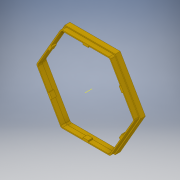
# Autodesk Inventor part: Cover v1
Saved by Autodesk Inventor 2019 (Build 230136000, 136)
## iProperties
Created: 2021-07-14
Part Number: Cover v1
Material: Generic
Document SubType Name: Modeling
Designer: Lix
Density: 1 g/cm^3
Appearance: Gold
d0: 175,000 mm
d1: 2,000 mm
d2: 0,00 deg
d15: 2,000 mm
d16: 2,000 mm
d17: 10,000 mm
d18: 0,00 deg
d19: 4,000 mm
d20: 7,000 mm
d21: 0,00 deg
d22: 10,000 mm
d23: 4,000 mm
d24: 10,000 mm
d25: 3,300 mm
d26: 6,500 mm
d27: 0,00 deg
d28: 4,000 mm
d29: 3,000 mm
d31: 0,00 deg
d32: 6,000 ul
d33: 360,00 deg
Author: Lix
Autodesk Inventor part; units mm, degrees
ref_plane "YZ Plane" through (0, 0, 0) normal (1, 0, 0) x (0, 1, 0)
ref_plane "XZ Plane" through (0, 0, 0) normal (0, 1, 0) x (-1, 0, 0)
ref_plane "XY Plane" through (0, 0, 0) normal (0, 0, 1) x (1, 0, 0)
sketch "Sketch1" plane through (0, 0, 0) normal (0, 0, 1) x (1, 0, 0)
  line L0 (50.5181, -87.5) -> (-50.5181, -87.5)
  line L1 (-50.5181, -87.5) -> (-101.0363, 0)
  line L2 (-101.0363, 0) -> (-50.5181, 87.5)
  line L3 (-50.5181, 87.5) -> (50.5181, 87.5)
  line L4 (50.5181, 87.5) -> (101.0363, 0)
  line L5 (101.0363, 0) -> (50.5181, -87.5)
  point P0 (0, 0)
  point P1 (0, 0)
  dimension "d0" = 175
  constraints: 12 end point, 1 coincident, 1 horizontal, 13 other
  measures "d0" distance between parallel lines of L4 L1
extrude "Extrusion1" add sketch "Sketch1" along normal blind 2
sketch "Sketch5" plane through (0, 0, 2) normal (0, 0, 1) x (1, 0, 0)
  line L0 (-50.5181, -87.5) -> (50.5181, -87.5) projected
  line L1 (50.5181, -87.5) -> (101.0363, 0) projected
  line L2 (101.0363, 0) -> (50.5181, 87.5) projected
  line L3 (50.5181, 87.5) -> (-50.5181, 87.5) projected
  line L4 (-50.5181, 87.5) -> (-101.0363, 0) projected
  line L5 (-101.0363, 0) -> (-50.5181, -87.5) projected
  line L6 (-98.7269, 0) -> (-49.3634, 85.5)
  line L7 (-49.3634, 85.5) -> (49.3634, 85.5)
  line L8 (49.3634, 85.5) -> (98.7269, 0)
  line L9 (98.7269, 0) -> (49.3634, -85.5)
  line L10 (49.3634, -85.5) -> (-49.3634, -85.5)
  line L11 (-49.3634, -85.5) -> (-98.7269, 0)
  line L12 (-96.4175, 0) -> (-48.2087, 83.5)
  line L13 (-48.2087, 83.5) -> (48.2087, 83.5)
  line L14 (48.2087, 83.5) -> (96.4175, 0)
  line L15 (96.4175, 0) -> (48.2087, -83.5)
  line L16 (48.2087, -83.5) -> (-48.2087, -83.5)
  line L17 (-48.2087, -83.5) -> (-96.4175, 0)
  point P0 (0, 0)
  dimension "d15" = 2
  dimension "d16" = 2
  constraints: 24 end point, 10 other
  measures "d15" distance between parallel lines of L4 L6
  measures "d16" distance between parallel lines of L11 L17
extrude "Extrusion5" add sketch "Sketch5" along normal blind 10 contours L6 L7 L8 L9 L10 L11
sketch "Sketch7" plane through (0, 0, 2) normal (0, 0, 1) x (1, 0, 0)
  line L0 (48.2087, 83.5) -> (-48.2087, 83.5) projected
  line L1 (-48.2087, 83.5) -> (-96.4175, 0) projected
  line L2 (-96.4175, 0) -> (-48.2087, -83.5) projected
  line L3 (-48.2087, -83.5) -> (48.2087, -83.5) projected
  line L4 (48.2087, -83.5) -> (96.4175, 0) projected
  line L5 (96.4175, 0) -> (48.2087, 83.5) projected
  line L6 (-45.8993, -79.5) -> (-91.7987, 0)
  line L7 (-91.7987, 0) -> (-45.8993, 79.5)
  line L8 (-45.8993, 79.5) -> (45.8993, 79.5)
  line L9 (45.8993, 79.5) -> (91.7987, 0)
  line L10 (91.7987, 0) -> (45.8993, -79.5)
  line L11 (45.8993, -79.5) -> (-45.8993, -79.5)
  point P0 (0, 0)
  dimension "d19" = 4
  constraints: 12 end point, 5 other
  measures "d19" distance between parallel lines of L2 L6
extrude "Extrusion6" cut sketch "Sketch7" against normal blind 7 contours L6 L7 L8 L9 L10 L11
fillet "Fillet1" radius 10 6 edges at (50.5181, 87.5, 1) (101.0363, 0, 1) (50.5181, -87.5, 1) (-50.5181, -87.5, 1) (-101.0363, 0, 1) (-50.5181, 87.5, 1)
fillet "Fillet1" radius 4 12 edges at (49.3634, -85.5, 7) (-48.2087, -83.5, 7) (-98.7269, 0, 7) (-49.3634, 85.5, 7) (49.3634, 85.5, 7) (98.7269, 0, 7) (48.2087, -83.5, 7) (96.4175, 0, 7) (-48.2087, 83.5, 7) (48.2087, 83.5, 7) (-49.3634, -85.5, 7) (-96.4175, 0, 7)
fillet "Fillet2" radius 10 6 edges at (45.8993, -79.5, 1) (91.7987, 0, 1) (45.8993, 79.5, 1) (-45.8993, 79.5, 1) (-91.7987, 0, 1) (-45.8993, -79.5, 1)
sketch "Sketch8" plane through (0, 0, 12) normal (0, 0, 1) x (1, 0, 0)
  line L0 (-1.65, 83.5) -> (1.65, 83.5)
  line L1 (1.65, 83.5) -> (1.65, 85.5)
  line L2 (1.65, 85.5) -> (-1.65, 85.5)
  line L3 (-1.65, 85.5) -> (-1.65, 83.5)
  line L4 (47.054, 85.5) -> (-47.054, 85.5) projected
  line L5 (-45.8993, 83.5) -> (45.8993, 83.5) projected
  point P0 (0, 0)
  point P1 (0, 85.5)
  point P2 (0, 85.5)
  point P3 (0, 0)
  dimension "d25" = 3.3
  constraints: 8 end point, 2 coincident, 2 collinear, 2 midpoint, 2 parallel, 1 horizontal, 1 perpendicular
  measures "d25" distance between parallel lines of L1 L3
extrude "Extrusion7" cut sketch "Sketch8" against normal blind 6.5
sketch "Sketch9" plane through (0, 0, 12) normal (0, 0, 1) x (1, 0, 0)
  line L0 (-4.65, 81.5) -> (-1.65, 81.5)
  line L1 (-1.65, 81.5) -> (-1.65, 85.5)
  line L2 (-1.65, 85.5) -> (-4.65, 85.5)
  line L3 (-4.65, 85.5) -> (-4.65, 81.5)
  line L4 (1.65, 83.5) -> (-1.65, 83.5) projected
  line L5 (1.65, 85.5) -> (1.65, 83.5) projected
  line L6 (-1.65, 85.5) -> (1.65, 85.5) projected
  line L7 (-1.65, 83.5) -> (-1.65, 85.5) projected
  line L8 (0, 83.5) -> (0, 81.6202) construction
  line L9 (-45.8993, 83.5) -> (-1.65, 83.5) projected
  line L10 (-1.65, 83.5) -> (-1.65, 85.5) projected
  line L11 (4.65, 81.5) -> (1.65, 81.5)
  line L12 (1.65, 81.5) -> (1.65, 85.5)
  line L13 (1.65, 85.5) -> (4.65, 85.5)
  line L14 (4.65, 85.5) -> (4.65, 81.5)
  line L15 (-1.65, 85.5) -> (-47.054, 85.5) projected
  point P0 (0, 0)
  dimension "d28" = 4
  dimension "d29" = 3
  constraints: 18 end point, 5 symmetric about line, 2 collinear, 2 parallel, 1 horizontal, 1 midpoint, 1 perpendicular, 1 vertical
  measures "d28" distance of L2.end L0.start
  measures "d29" distance of L1.end L2.end
extrude "Extrusion8" add sketch "Sketch9" against normal up to surface (10 mm away) contours L3 L9 L1 L0 | L3 L2 L1 L9 | L5 L13 L14 L11 L12
pattern_circular "Circular Pattern1" count 6 over 360 about axis through (0, 0, 0) along (0, 0, 1) of "Extrusion8", "Extrusion7"
sketch "Sketch11" plane through (0, 0, 0) normal (0, 0, -1) x (-1, 0, 0)
  arc A0 (53.4049, 82.5) -> (44.7446, 87.5) centre (44.7446, 77.5) ccw projected
  line L0 (44.7446, 87.5) -> (-44.7446, 87.5) projected
  arc A1 (-44.7446, 87.5) -> (-53.4049, 82.5) centre (-44.7446, 77.5) ccw projected
  line L1 (-53.4049, 82.5) -> (-98.1495, 5) projected
  arc A2 (-98.1495, 5) -> (-98.1495, -5) centre (-89.4893, 0) ccw projected
  line L2 (-98.1495, -5) -> (-53.4049, -82.5) projected
  arc A3 (-53.4049, -82.5) -> (-44.7446, -87.5) centre (-44.7446, -77.5) ccw projected
  line L3 (-44.7446, -87.5) -> (44.7446, -87.5) projected
  arc A4 (44.7446, -87.5) -> (53.4049, -82.5) centre (44.7446, -77.5) ccw projected
  line L4 (53.4049, -82.5) -> (98.1495, -5) projected
  arc A5 (98.1495, -5) -> (98.1495, 5) centre (89.4893, 0) ccw projected
  line L5 (98.1495, 5) -> (53.4049, 82.5) projected
  line L6 (40.1258, -79.5) -> (-40.1258, -79.5) projected
  arc A6 (-48.7861, -74.5) -> (-40.1258, -79.5) centre (-40.1258, -69.5) ccw projected
  line L7 (-48.7861, -74.5) -> (-88.9119, -5) projected
  arc A7 (-88.9119, 5) -> (-88.9119, -5) centre (-80.2517, 0) ccw projected
  line L8 (-88.9119, 5) -> (-48.7861, 74.5) projected
  arc A8 (-40.1258, 79.5) -> (-48.7861, 74.5) centre (-40.1258, 69.5) ccw projected
  line L9 (-40.1258, 79.5) -> (40.1258, 79.5) projected
  arc A9 (48.7861, 74.5) -> (40.1258, 79.5) centre (40.1258, 69.5) ccw projected
  line L10 (48.7861, 74.5) -> (88.9119, 5) projected
  arc A10 (88.9119, -5) -> (88.9119, 5) centre (80.2517, 0) ccw projected
  line L11 (88.9119, -5) -> (48.7861, -74.5) projected
  arc A11 (40.1258, -79.5) -> (48.7861, -74.5) centre (40.1258, -69.5) ccw projected
  point P0 (0, 0)
extrude "Extrusion9" cut sketch "Sketch11" against normal blind 3
sketch "Sketch12" plane through (0, 0, 12) normal (0, 0, 1) x (1, 0, 0)
  line L0 (74.6381, 37.723) -> (95.2628, 2) projected
  arc A0 (95.2628, -2) -> (95.2628, 2) centre (91.7987, 0) ccw projected
  line L1 (95.2628, -2) -> (74.6381, -37.723) projected
  line L2 (74.6381, -37.723) -> (72.9061, -36.723) projected
  line L3 (72.9061, -36.723) -> (71.4061, -39.3211) projected
  line L4 (71.4061, -39.3211) -> (74.8702, -41.3211) projected
  line L5 (74.8702, -41.3211) -> (97.5722, -2) projected
  arc A1 (97.5722, -2) -> (97.5722, 2) centre (94.1081, 0) ccw projected
  line L6 (97.5722, 2) -> (74.8702, 41.3211) projected
  line L7 (71.4061, 39.3211) -> (74.8702, 41.3211) projected
  line L8 (72.9061, 36.723) -> (71.4061, 39.3211) projected
  line L9 (74.6381, 37.723) -> (72.9061, 36.723) projected
  line L10 (73.2202, 44.1789) -> (50.5181, 83.5) projected
  arc A2 (50.5181, 83.5) -> (47.054, 85.5) centre (47.054, 81.5) ccw projected
  line L11 (47.054, 85.5) -> (1.65, 85.5) projected
  line L12 (1.65, 81.5) -> (1.65, 85.5) projected
  line L13 (4.65, 81.5) -> (1.65, 81.5) projected
  line L14 (4.65, 83.5) -> (4.65, 81.5) projected
  line L15 (4.65, 83.5) -> (45.8993, 83.5) projected
  arc A3 (49.3634, 81.5) -> (45.8993, 83.5) centre (45.8993, 79.5) ccw projected
  line L16 (49.3634, 81.5) -> (69.9881, 45.777) projected
  line L17 (69.9881, 45.777) -> (68.2561, 44.777) projected
  line L18 (68.2561, 44.777) -> (69.7561, 42.1789) projected
  line L19 (69.7561, 42.1789) -> (73.2202, 44.1789) projected
  line L20 (-69.9881, 45.777) -> (-49.3634, 81.5) projected
  arc A4 (-45.8993, 83.5) -> (-49.3634, 81.5) centre (-45.8993, 79.5) ccw projected
  line L21 (-45.8993, 83.5) -> (-4.65, 83.5) projected
  line L22 (-4.65, 83.5) -> (-4.65, 81.5) projected
  line L23 (-4.65, 81.5) -> (-1.65, 81.5) projected
  line L24 (-1.65, 81.5) -> (-1.65, 85.5) projected
  line L25 (-1.65, 85.5) -> (-47.054, 85.5) projected
  arc A5 (-47.054, 85.5) -> (-50.5181, 83.5) centre (-47.054, 81.5) ccw projected
  line L26 (-50.5181, 83.5) -> (-73.2202, 44.1789) projected
  line L27 (-69.7561, 42.1789) -> (-73.2202, 44.1789) projected
  line L28 (-68.2561, 44.777) -> (-69.7561, 42.1789) projected
  line L29 (-69.9881, 45.777) -> (-68.2561, 44.777) projected
  line L30 (-74.6381, -37.723) -> (-95.2628, -2) projected
  arc A6 (-95.2628, 2) -> (-95.2628, -2) centre (-91.7987, 0) ccw projected
  line L31 (-95.2628, 2) -> (-74.6381, 37.723) projected
  line L32 (-74.6381, 37.723) -> (-72.9061, 36.723) projected
  line L33 (-72.9061, 36.723) -> (-71.4061, 39.3211) projected
  line L34 (-71.4061, 39.3211) -> (-74.8702, 41.3211) projected
  line L35 (-74.8702, 41.3211) -> (-97.5722, 2) projected
  arc A7 (-97.5722, 2) -> (-97.5722, -2) centre (-94.1081, 0) ccw projected
  line L36 (-97.5722, -2) -> (-74.8702, -41.3211) projected
  line L37 (-71.4061, -39.3211) -> (-74.8702, -41.3211) projected
  line L38 (-72.9061, -36.723) -> (-71.4061, -39.3211) projected
  line L39 (-74.6381, -37.723) -> (-72.9061, -36.723) projected
  line L40 (-4.65, -83.5) -> (-45.8993, -83.5) projected
  arc A8 (-49.3634, -81.5) -> (-45.8993, -83.5) centre (-45.8993, -79.5) ccw projected
  line L41 (-49.3634, -81.5) -> (-69.9881, -45.777) projected
  line L42 (-69.9881, -45.777) -> (-68.2561, -44.777) projected
  line L43 (-68.2561, -44.777) -> (-69.7561, -42.1789) projected
  line L44 (-69.7561, -42.1789) -> (-73.2202, -44.1789) projected
  line L45 (-73.2202, -44.1789) -> (-50.5181, -83.5) projected
  arc A9 (-50.5181, -83.5) -> (-47.054, -85.5) centre (-47.054, -81.5) ccw projected
  line L46 (-47.054, -85.5) -> (-1.65, -85.5) projected
  line L47 (-1.65, -81.5) -> (-1.65, -85.5) projected
  line L48 (-4.65, -81.5) -> (-1.65, -81.5) projected
  line L49 (-4.65, -83.5) -> (-4.65, -81.5) projected
  line L50 (69.9881, -45.777) -> (49.3634, -81.5) projected
  arc A10 (45.8993, -83.5) -> (49.3634, -81.5) centre (45.8993, -79.5) ccw projected
  line L51 (45.8993, -83.5) -> (4.65, -83.5) projected
  line L52 (4.65, -83.5) -> (4.65, -81.5) projected
  line L53 (4.65, -81.5) -> (1.65, -81.5) projected
  line L54 (1.65, -81.5) -> (1.65, -85.5) projected
  line L55 (1.65, -85.5) -> (47.054, -85.5) projected
  arc A11 (47.054, -85.5) -> (50.5181, -83.5) centre (47.054, -81.5) ccw projected
  line L56 (50.5181, -83.5) -> (73.2202, -44.1789) projected
  line L57 (69.7561, -42.1789) -> (73.2202, -44.1789) projected
  line L58 (68.2561, -44.777) -> (69.7561, -42.1789) projected
  line L59 (69.9881, -45.777) -> (68.2561, -44.777) projected
  line L60 (74.6381, 37.723) -> (72.9061, 36.723) projected
  line L61 (72.9061, 36.723) -> (76.3702, 38.723)
  line L62 (97.5722, 2) -> (74.8702, 41.3211) projected
  line L63 (76.3702, 38.723) -> (74.8702, 41.3211)
  line L64 (74.8702, 41.3211) -> (71.4061, 39.3211)
  line L65 (71.4061, 39.3211) -> (72.9061, 36.723)
  line L66 (69.7561, 42.1789) -> (73.2202, 44.1789) projected
  line L67 (73.2202, 44.1789) -> (69.7561, 42.1789)
  line L68 (69.7561, 42.1789) -> (68.2561, 44.777)
  line L69 (68.2561, 44.777) -> (71.7202, 46.777)
  line L70 (71.7202, 46.777) -> (73.2202, 44.1789)
  line L71 (97.5722, 2) -> (50.5181, 83.5) projected
  point P0 (0, 0)
  constraints: 16 end point, 6 perpendicular, 2 collinear, 2 point on line
extrude "Extrusion10" cut sketch "Sketch12" against normal blind 3 contours L19 L18 L17 L69 L10 | L9 L8 L7 L6 L61
sketch "Sketch13" plane through (73.1381, 40.3211, 5.5) normal (0, 0, 1) x (0.866, 0.5, 0)
  line L0 (0, 0) -> (0, 3.3) projected
  line L1 (2, 0) -> (0, 0) projected
  line L2 (2, 3.3) -> (2, 0) projected
  line L3 (0, 3.3) -> (2, 3.3) projected
  line L4 (2, 6.3) -> (2, 3.3) projected
  line L5 (0, 6.3) -> (2, 6.3) projected
  line L6 (-2, 6.3) -> (0, 6.3) projected
  line L7 (-2, 3.3) -> (-2, 6.3) projected
  line L8 (2, 3.3) -> (-2, 3.3) projected
  line L9 (2, -3) -> (0, -3) projected
  line L10 (2, 0) -> (2, -3) projected
  line L11 (-2, 0) -> (2, 0) projected
  line L12 (-2, -3) -> (-2, 0) projected
  line L13 (0, -3) -> (-2, -3) projected
  line L14 (0, 0) -> (-2, 0) projected
  line L15 (2, 3.3) -> (-2, 3.3)
  line L16 (-2, 3.3) -> (-2, 0)
  line L17 (-2, 0) -> (2, 0)
  line L18 (2, 0) -> (2, 3.3)
  point P0 (-83.5, 1.65)
  constraints: 8 end point, 2 parallel, 1 horizontal, 1 perpendicular
extrude "Extrusion11" add sketch "Sketch13" along normal blind 3.5 contours L11 L16 L8 L0 | L0 L3 L2 L1
pattern_circular "Circular Pattern2" count 6 over 360 about axis through (0, 0, 0) along (0, 0, 1) of "Extrusion11", "Extrusion10"
sketch "Sketch14" plane through (0, 0, 3) normal (0, 0, -1) x (-1, 0, 0)
  line L0 (1.65, 83.5) -> (-1.65, 83.5) projected
  line L1 (1.65, 81.5) -> (1.65, 83.5) projected
  line L2 (4.65, 81.5) -> (1.65, 81.5) projected
  line L3 (4.65, 83.5) -> (4.65, 81.5) projected
  line L4 (45.8993, 83.5) -> (4.65, 83.5) projected
  arc A0 (49.3634, 81.5) -> (45.8993, 83.5) centre (45.8993, 79.5) ccw projected
  line L5 (69.9881, 45.777) -> (49.3634, 81.5) projected
  line L6 (68.2561, 44.777) -> (69.9881, 45.777) projected
  line L7 (69.7561, 42.1789) -> (68.2561, 44.777) projected
  line L8 (71.4881, 43.1789) -> (69.7561, 42.1789) projected
  line L9 (73.1381, 40.3211) -> (71.4881, 43.1789) projected
  line L10 (71.4061, 39.3211) -> (73.1381, 40.3211) projected
  line L11 (72.9061, 36.723) -> (71.4061, 39.3211) projected
  line L12 (74.6381, 37.723) -> (72.9061, 36.723) projected
  line L13 (95.2628, 2) -> (74.6381, 37.723) projected
  arc A1 (95.2628, -2) -> (95.2628, 2) centre (91.7987, 0) ccw projected
  line L14 (74.6381, -37.723) -> (95.2628, -2) projected
  line L15 (72.9061, -36.723) -> (74.6381, -37.723) projected
  line L16 (71.4061, -39.3211) -> (72.9061, -36.723) projected
  line L17 (73.1381, -40.3211) -> (71.4061, -39.3211) projected
  line L18 (71.4881, -43.1789) -> (73.1381, -40.3211) projected
  line L19 (69.7561, -42.1789) -> (71.4881, -43.1789) projected
  line L20 (68.2561, -44.777) -> (69.7561, -42.1789) projected
  line L21 (69.9881, -45.777) -> (68.2561, -44.777) projected
  line L22 (49.3634, -81.5) -> (69.9881, -45.777) projected
  arc A2 (45.8993, -83.5) -> (49.3634, -81.5) centre (45.8993, -79.5) ccw projected
  line L23 (4.65, -83.5) -> (45.8993, -83.5) projected
  line L24 (4.65, -81.5) -> (4.65, -83.5) projected
  line L25 (1.65, -81.5) -> (4.65, -81.5) projected
  line L26 (1.65, -83.5) -> (1.65, -81.5) projected
  line L27 (-1.65, -83.5) -> (1.65, -83.5) projected
  line L28 (-1.65, -81.5) -> (-1.65, -83.5) projected
  line L29 (-4.65, -81.5) -> (-1.65, -81.5) projected
  line L30 (-4.65, -83.5) -> (-4.65, -81.5) projected
  line L31 (-45.8993, -83.5) -> (-4.65, -83.5) projected
  arc A3 (-49.3634, -81.5) -> (-45.8993, -83.5) centre (-45.8993, -79.5) ccw projected
  line L32 (-69.9881, -45.777) -> (-49.3634, -81.5) projected
  line L33 (-68.2561, -44.777) -> (-69.9881, -45.777) projected
  line L34 (-69.7561, -42.1789) -> (-68.2561, -44.777) projected
  line L35 (-71.4881, -43.1789) -> (-69.7561, -42.1789) projected
  line L36 (-73.1381, -40.3211) -> (-71.4881, -43.1789) projected
  line L37 (-71.4061, -39.3211) -> (-73.1381, -40.3211) projected
  line L38 (-72.9061, -36.723) -> (-71.4061, -39.3211) projected
  line L39 (-74.6381, -37.723) -> (-72.9061, -36.723) projected
  line L40 (-95.2628, -2) -> (-74.6381, -37.723) projected
  arc A4 (-95.2628, 2) -> (-95.2628, -2) centre (-91.7987, 0) ccw projected
  line L41 (-74.6381, 37.723) -> (-95.2628, 2) projected
  line L42 (-72.9061, 36.723) -> (-74.6381, 37.723) projected
  line L43 (-71.4061, 39.3211) -> (-72.9061, 36.723) projected
  line L44 (-73.1381, 40.3211) -> (-71.4061, 39.3211) projected
  line L45 (-71.4881, 43.1789) -> (-73.1381, 40.3211) projected
  line L46 (-69.7561, 42.1789) -> (-71.4881, 43.1789) projected
  line L47 (-68.2561, 44.777) -> (-69.7561, 42.1789) projected
  line L48 (-69.9881, 45.777) -> (-68.2561, 44.777) projected
  line L49 (-49.3634, 81.5) -> (-69.9881, 45.777) projected
  arc A5 (-45.8993, 83.5) -> (-49.3634, 81.5) centre (-45.8993, 79.5) ccw projected
  line L50 (-4.65, 83.5) -> (-45.8993, 83.5) projected
  line L51 (-4.65, 81.5) -> (-4.65, 83.5) projected
  line L52 (-1.65, 81.5) -> (-4.65, 81.5) projected
  line L53 (-1.65, 83.5) -> (-1.65, 81.5) projected
  line L54 (-47.054, 85.5) -> (47.054, 85.5) projected
  arc A6 (-47.054, 85.5) -> (-50.5181, 83.5) centre (-47.054, 81.5) ccw projected
  line L55 (-97.5722, 2) -> (-50.5181, 83.5) projected
  arc A7 (-97.5722, 2) -> (-97.5722, -2) centre (-94.1081, 0) ccw projected
  line L56 (-50.5181, -83.5) -> (-97.5722, -2) projected
  arc A8 (-50.5181, -83.5) -> (-47.054, -85.5) centre (-47.054, -81.5) ccw projected
  line L57 (47.054, -85.5) -> (-47.054, -85.5) projected
  arc A9 (47.054, -85.5) -> (50.5181, -83.5) centre (47.054, -81.5) ccw projected
  line L58 (97.5722, -2) -> (50.5181, -83.5) projected
  arc A10 (97.5722, -2) -> (97.5722, 2) centre (94.1081, 0) ccw projected
  line L59 (50.5181, 83.5) -> (97.5722, 2) projected
  arc A11 (50.5181, 83.5) -> (47.054, 85.5) centre (47.054, 81.5) ccw projected
  line L60 (5.35, -85.5) -> (-5.35, -85.5)
  line L61 (-5.35, -85.5) -> (-5.35, -80.8)
  line L62 (-5.35, -80.8) -> (5.35, -80.8)
  line L63 (5.35, -80.8) -> (5.35, -85.5)
  point P0 (0, 0)
  dimension "d44" = 0.7
  dimension "d45" = 0.7
  dimension "d46" = 0.7
  constraints: 8 end point, 2 parallel, 1 collinear, 1 horizontal, 1 perpendicular
  measures "d44" distance between parallel lines of L63 L24
  measures "d45" distance between parallel lines of L30 L61
  measures "d46" distance between parallel lines of L62 L29
extrude "Extrusion12" add sketch "Sketch14" against normal up to surface (9 mm away) contours L63 L57 L61 L31 L30 L29 L28 L27 L26 L25 L24 L23 | L23 L24 L25 L26 L27 L28 L29 L30 L31 L61 L62 L63
pattern_circular "Circular Pattern3" count 6 over 360 about axis through (0, 0, 0) along (0, 0, 1) of "Extrusion12"
sketch "Sketch15" plane through (0, 0, 3) normal (0, 0, -1) x (-1, 0, 0)
  line L0 (49.3634, -81.5) -> (69.6381, -46.3832) projected
  arc A0 (45.8993, -83.5) -> (49.3634, -81.5) centre (45.8993, -79.5) ccw projected
  line L1 (5.35, -83.5) -> (45.8993, -83.5) projected
  line L2 (5.35, -80.8) -> (5.35, -83.5) projected
  line L3 (-5.35, -80.8) -> (5.35, -80.8) projected
  line L4 (-5.35, -83.5) -> (-5.35, -80.8) projected
  line L5 (-45.8993, -83.5) -> (-5.35, -83.5) projected
  arc A1 (-49.3634, -81.5) -> (-45.8993, -83.5) centre (-45.8993, -79.5) ccw projected
  line L6 (-69.6381, -46.3832) -> (-49.3634, -81.5) projected
  line L7 (-67.2999, -45.0332) -> (-69.6381, -46.3832) projected
  line L8 (-72.6499, -35.7668) -> (-67.2999, -45.0332) projected
  line L9 (-74.9881, -37.1168) -> (-72.6499, -35.7668) projected
  line L10 (-95.2628, -2) -> (-74.9881, -37.1168) projected
  arc A2 (-95.2628, 2) -> (-95.2628, -2) centre (-91.7987, 0) ccw projected
  line L11 (-74.9881, 37.1168) -> (-95.2628, 2) projected
  line L12 (-72.6499, 35.7668) -> (-74.9881, 37.1168) projected
  line L13 (-67.2999, 45.0332) -> (-72.6499, 35.7668) projected
  line L14 (-69.6381, 46.3832) -> (-67.2999, 45.0332) projected
  line L15 (-49.3634, 81.5) -> (-69.6381, 46.3832) projected
  arc A3 (-45.8993, 83.5) -> (-49.3634, 81.5) centre (-45.8993, 79.5) ccw projected
  line L16 (-5.35, 83.5) -> (-45.8993, 83.5) projected
  line L17 (-5.35, 80.8) -> (-5.35, 83.5) projected
  line L18 (5.35, 80.8) -> (-5.35, 80.8) projected
  line L19 (5.35, 83.5) -> (5.35, 80.8) projected
  line L20 (45.8993, 83.5) -> (5.35, 83.5) projected
  arc A4 (49.3634, 81.5) -> (45.8993, 83.5) centre (45.8993, 79.5) ccw projected
  line L21 (69.6381, 46.3832) -> (49.3634, 81.5) projected
  line L22 (67.2999, 45.0332) -> (69.6381, 46.3832) projected
  line L23 (72.6499, 35.7668) -> (67.2999, 45.0332) projected
  line L24 (74.9881, 37.1168) -> (72.6499, 35.7668) projected
  line L25 (95.2628, 2) -> (74.9881, 37.1168) projected
  arc A5 (95.2628, -2) -> (95.2628, 2) centre (91.7987, 0) ccw projected
  line L26 (74.9881, -37.1168) -> (95.2628, -2) projected
  line L27 (72.6499, -35.7668) -> (74.9881, -37.1168) projected
  line L28 (67.2999, -45.0332) -> (72.6499, -35.7668) projected
  line L29 (69.6381, -46.3832) -> (67.2999, -45.0332) projected
  line L30 (97.5722, -2) -> (50.5181, -83.5) projected
  arc A6 (97.5722, -2) -> (97.5722, 2) centre (94.1081, 0) ccw projected
  line L31 (50.5181, 83.5) -> (97.5722, 2) projected
  arc A7 (50.5181, 83.5) -> (47.054, 85.5) centre (47.054, 81.5) ccw projected
  line L32 (-47.054, 85.5) -> (47.054, 85.5) projected
  arc A8 (-47.054, 85.5) -> (-50.5181, 83.5) centre (-47.054, 81.5) ccw projected
  line L33 (-97.5722, 2) -> (-50.5181, 83.5) projected
  arc A9 (-97.5722, 2) -> (-97.5722, -2) centre (-94.1081, 0) ccw projected
  line L34 (-50.5181, -83.5) -> (-97.5722, -2) projected
  arc A10 (-50.5181, -83.5) -> (-47.054, -85.5) centre (-47.054, -81.5) ccw projected
  line L35 (47.054, -85.5) -> (-47.054, -85.5) projected
  arc A11 (47.054, -85.5) -> (50.5181, -83.5) centre (47.054, -81.5) ccw projected
  line L36 (-50.5181, -87.5) -> (-101.0363, 0)
  line L37 (-101.0363, 0) -> (-50.5181, 87.5)
  line L38 (-50.5181, 87.5) -> (50.5181, 87.5)
  line L39 (50.5181, 87.5) -> (101.0363, 0)
  line L40 (101.0363, 0) -> (50.5181, -87.5)
  line L41 (50.5181, -87.5) -> (-50.5181, -87.5)
  point P0 (0, 0)
  point P1 (0, 0)
  dimension "d52" = 175
  constraints: 12 end point, 1 coincident, 1 parallel, 13 other
  measures "d52" distance between parallel lines of L36 L39
extrude "Extrusion13" add sketch "Sketch15" along normal blind 10 contours L36 L37 L38 L39 L40 L41
equation "\"d45\" = d44"
equation "\"d46\" = d44"
body "Solid1"
